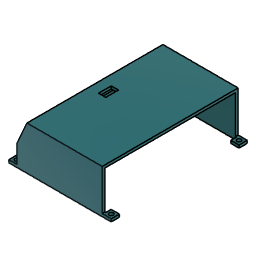
PerryBot (Autodesk Fusion 360 archive; units mm, degrees)
design "PerryBot2_Lid"
Autodesk Fusion 360 part; units mm, degrees
sketch "Sketch1" plane through (0, 0, 0) normal (0, 0, 1) x (1, 0, 0)
  line L0 (56.5, 75) -> (-56.5, 75)
  line L1 (-56.5, 75) -> (-56.5, -75)
  line L2 (-56.5, -75) -> (56.5, -75)
  line L3 (56.5, -75) -> (56.5, 75)
  line L4 (56.5, 75) -> (-56.5, -75) construction
  line L5 (-56.5, 75) -> (56.5, -75) construction
  line L6 (47.5, 75) -> (47.5, -75)
  line L7 (47.5, 66) -> (56.5, 66)
  line L8 (56.5, -66) -> (47.5, -66)
  dimension "d1" = 113
  dimension "d2" = 150
  dimension "d5" = 104
  dimension "d43" = 9
  dimension "d45" = 9
  constraint horizontal L0
  constraint perpendicular L0 L1
  constraint parallel L0 L2
  constraint parallel L1 L3
  constraint coincident L4 origin
  constraint coincident L5 origin
  constraint coincident L0 L6.start
  constraint coincident L2 L6.end
  constraint perpendicular L2 L6
  constraint coincident L6 L7.start
  constraint coincident L3 L7.end
  constraint perpendicular L6 L7
  constraint coincident L3 L8.start
  constraint coincident L6 L8.end
  constraint perpendicular L6 L8
  measures "d1" distance of L0.start L0.end
  measures "d2" distance of L0.start L2.end
  measures "d5" distance of L1 L6
  measures "d43" distance of L0 L7
  measures "d45" distance of L2 L8
extrude "Extrude1" add sketch "Sketch1" along normal blind 3 contours L0 L3 L6 L7 | L0 L1 L2 L6 | L2 L3 L6 L8 makes body 1
sketch "Sketch2" plane through (0, 0, 3) normal (0, 0, 1) x (-1, 0, 0)
  line L0 (-56.5, -66) -> (-56.5, -75)
  line L1 (-56.5, -75) -> (56.5, -75)
  line L2 (56.5, -75) -> (56.5, 75)
  line L3 (56.5, 75) -> (-56.5, 75)
  circle A0 centre (52, -70.5) radius 2.25
  line L4 (52, -70.5) -> (52, -75) construction
  line L5 (52, -70.5) -> (56.5, -70.5) construction
  line L6 (56.5, -75) -> (47.5, -75)
  line L7 (47.5, -75) -> (47.5, -66)
  line L8 (47.5, -66) -> (56.5, -66)
  line L9 (56.5, -66) -> (56.5, -75)
  line L10 (56.5, -75) -> (47.5, -66) construction
  line L11 (47.5, -75) -> (56.5, -66) construction
  line L12 (-47.5, -66) -> (-56.5, -66)
  line L13 (-56.5, 75) -> (-56.5, 66)
  line L14 (-56.5, 66) -> (-47.5, 66)
  line L15 (-47.5, 66) -> (-47.5, -66)
  point P0 (52, -70.5)
  dimension "d8" = 4.5
  dimension "d10" = 4.5
  constraint coincident P0 A0.centre
  constraint coincident L1 L4.end
  constraint perpendicular L1 L4
  constraint coincident L2 L5.end
  constraint perpendicular L2 L5
  constraint equal L4 L5
  constraint horizontal L6
  constraint perpendicular L6 L7
  constraint parallel L6 L8
  constraint parallel L7 L9
  constraint coincident L10 P0
  constraint coincident L11 P0
  constraint coincident L1.end L2.start
  measures "d8" diameter of A0
  measures "d10" distance of P0 L4.end
ref_plane "WorkPlane1" through (0, 0, 1.5) normal (0, 1, 0) x (-1, 0, 0)
ref_plane "WorkPlane2" through (0, 0, 1.5) normal (-1, 0, 0) x (0, -1, 0)
extrude "Extrude2" cut sketch "Sketch2" against normal blind 3 contours A0 bodies 1
mirror "Mirror1" about plane through (0, 0, 1.5) normal (-1, 0, 0) of "Extrude2"
mirror "Mirror2" about plane through (0, 0, 1.5) normal (0, 1, 0) of "Extrude2", "Mirror1"
ref_plane "WorkPlane3" through (0, -75, 1.5) normal (0, -1, 0) x (1, 0, 0)
sketch "Sketch5" plane through (0, -75, 0) normal (0, -1, 0) x (-1, 0, 0)
  line L0 (56.5, -3) -> (36.5, -3) construction
  line L1 (36.5, -3) -> (36.5, -48) construction
  line L2 (56.5, -3) -> (56.5, 0) construction
  line L3 (36.5, -48) -> (56.5, -3)
  line L4 (36.5, -48) -> (-46.5, -48)
  line L5 (-46.5, -48) -> (-46.5, -3)
  line L6 (-46.5, -3) -> (56.5, -3)
  line L7 (23, -104) -> (21.5469, -104)
  point P0 (56.5, 0)
  dimension "d32" = 20
  dimension "d33" = 45
  dimension "d34" = 3
  dimension "d36" = 83
  constraint horizontal L0
  constraint perpendicular L0 L1
  constraint coincident P0 L2.end
  constraint vertical L2
  constraint perpendicular L1 L4
  constraint perpendicular L0 L5
  constraint parallel L0 L6
  constraint perpendicular L5 L7
  measures "d32" distance of L0.start L0.end
  measures "d33" distance of L0.end L1.end
  measures "d34" distance of L0.start P0
  measures "d36" distance of L1.end L4.end
extrude "Extrude5" add sketch "Sketch5" against normal up to surface (150 mm away) separate body makes body 2
extrude "Extrude6" cut sketch "Sketch2" along normal blind 45 contours L1 L2 L6 L7 L8 L9 | A0 bodies 2
mirror "Mirror3" about plane through (0, 0, 1.5) normal (0, 1, 0) of "Extrude6"
sketch "Sketch7" plane through (46.5, 0, 0) normal (1, 0, 0) x (0, 1, 0)
  line L0 (75, 3) -> (75, 48)
  line L1 (75, 48) -> (-75, 48)
  line L2 (-75, 48) -> (-75, 3)
  line L3 (-75, 3) -> (75, 3)
  line L4 (-66, 0) -> (-72, 0)
  line L5 (-72, 0) -> (-72, 3)
  line L6 (-72, 3) -> (-66, 3)
  line L7 (-66, 3) -> (-66, 0)
  line L8 (-72, 3) -> (-72, 45)
  line L9 (-72, 45) -> (72, 45)
  line L10 (72, 45) -> (72, 3)
  dimension "d47" = 3
  dimension "d48" = 3
  dimension "d49" = 3
  constraint horizontal L4
  constraint vertical L5
  constraint horizontal L6
  constraint vertical L7
  constraint coincident L3 L5.end
  constraint perpendicular L6 L8
  constraint perpendicular L8 L9
  constraint coincident L3 L10.end
  constraint perpendicular L3 L10
  measures "d47" distance of L2.end L5.end
  measures "d48" distance of L1 L8.end
  measures "d49" distance of L0 L9.end
extrude "Extrude7" cut sketch "Sketch7" 1 faces at (47.5, 22, 1) against normal blind 83 contours L3 L6 L8 L9 L10 on bodies 1 bodies 1 2
sketch "Sketch8" plane through (0, 0, 3) normal (0, 0, 1) x (-1, 0, 0)
  circle A0 centre (52, -70.5) radius 2.25
  circle A1 centre (-52, -70.5) radius 2.25
  circle A2 centre (52, 70.5) radius 2.25
  circle A3 centre (-52, 70.5) radius 2.25
  line L0 (35.5, -66) -> (-56.5, -66)
  line L1 (-56.5, -66) -> (-56.5, -75)
  line L2 (-56.5, -75) -> (56.5, -75)
  line L3 (56.5, -75) -> (56.5, 75)
  line L4 (56.5, 75) -> (-56.5, 75)
  line L5 (-56.5, 75) -> (-56.5, 66)
  line L6 (-56.5, 66) -> (35.5, 66)
  line L7 (35.5, 66) -> (35.5, -66)
  line L8 (-47.5, 72) -> (-47.5, 66)
  line L9 (-47.5, 72) -> (35.5, 72)
  line L10 (35.5, 72) -> (35.5, 66)
  line L11 (-47.5, 66) -> (35.5, 66)
  line L12 (36.5, 72) -> (-46.5, 72)
  dimension "d52" = 9
  constraint coincident L6 L8.end
  constraint perpendicular L6 L8
  constraint perpendicular L3 L9
  constraint coincident L6.end L7.start
  constraint collinear L7 L10
  constraint collinear L9 L12
  measures "d52" distance of L5 L8
extrude "Extrude8" cut sketch "Sketch8" against normal up to surface (3 mm away) contours L6 L8 L9 L10 L11 L12 bodies 1
mirror "Mirror4" about plane through (0, 0, 1.5) normal (0, 1, 0) of "Extrude8"
sketch "Sketch9" plane through (0, -75, 0) normal (0, -1, 0) x (1, 0, 0)
  line L0 (-47.5, 23.25) -> (-47.5, 3)
  line L1 (-47.5, 3) -> (46.5, 3)
  line L2 (46.5, 3) -> (46.5, 48)
  line L3 (46.5, 48) -> (-36.5, 48)
  line L4 (-36.5, 48) -> (-47.5, 23.25)
  line L5 (-45.5, 3) -> (-45.5, 22.8256)
  line L6 (-45.5, 22.8256) -> (-36.5, 43.0756)
  line L7 (-41.3061, 32.2618) -> (-43.1338, 33.074) construction
  line L8 (-45.5, 16.8092) -> (-47.5, 16.8092) construction
  line L9 (-36.5, 43.0756) -> (-36.5, 3)
  dimension "d60" = 2
  constraint coincident L1 L5.start
  constraint perpendicular L1 L5
  constraint parallel L4 L6
  constraint vertical L3.end L6.end
  constraint coincident L6 L7.start
  constraint coincident L4 L7.end
  constraint perpendicular L4 L7
  constraint coincident L5 L8.start
  constraint coincident L0 L8.end
  constraint perpendicular L0 L8
  constraint equal L7 L8
  constraint coincident L1 L9.end
  constraint perpendicular L1 L9
  measures "d60" distance of L0 L5
extrude "Extrude9" cut sketch "Sketch9" against normal up to surface (144 mm away) from surface at -3 contours L1 L5 L6 L9 bodies 2
sketch "Sketch10" plane through (0, 0, 3) normal (0, 0, 1) x (-1, 0, 0)
  circle A0 centre (52, -70.5) radius 2.25
  circle A1 centre (-52, -70.5) radius 2.25
  circle A2 centre (52, 70.5) radius 2.25
  circle A3 centre (-52, 70.5) radius 2.25
  line L0 (35.5, 72) -> (35.5, -72)
  line L1 (35.5, -72) -> (-47.5, -72)
  line L2 (-47.5, -72) -> (-47.5, -66)
  line L3 (-47.5, -66) -> (-56.5, -66)
  line L4 (-56.5, -66) -> (-56.5, -75)
  line L5 (-56.5, -75) -> (56.5, -75)
  line L6 (56.5, -75) -> (56.5, 75)
  line L7 (56.5, 75) -> (-56.5, 75)
  line L8 (-56.5, 75) -> (-56.5, 66)
  line L9 (-56.5, 66) -> (-47.5, 66)
  line L10 (-47.5, 66) -> (-47.5, 72)
  line L11 (-47.5, 72) -> (35.5, 72)
  line L12 (35.5, 72) -> (45.5, 72)
  line L13 (45.5, 72) -> (45.5, -72)
  line L14 (45.5, -72) -> (35.5, -72)
  line L15 (35.5, 72) -> (35.5, -72)
  line L16 (45.5, -72) -> (45.5, 72)
  constraint coincident L0.start L11.end
  constraint perpendicular L5 L13
  constraint coincident L0.end L1.start
  constraint parallel L1 L14
  constraint collinear L13 L16
extrude "Extrude10" cut sketch "Sketch10" against normal blind 3 contours L0 L12 L13 L14 L15 L16 bodies 1
combine "Combine1" operation add target body 1 tool bodies 2
sketch "Sketch11" plane through (0, 0, 48) normal (0, 0, 1) x (-1, 0, 0)
  line L0 (-46.5, -75) -> (36.5, -75)
  line L1 (36.5, -75) -> (36.5, 75)
  line L2 (36.5, 75) -> (-46.5, 75)
  line L3 (-46.5, 75) -> (-46.5, -75)
  line L4 (17.5, -7) -> (25.5, -7)
  line L5 (25.5, -7) -> (25.5, 7)
  line L6 (25.5, 7) -> (17.5, 7)
  line L7 (17.5, 7) -> (17.5, -7)
  line L8 (17.5, -7) -> (25.5, 7) construction
  line L9 (25.5, -7) -> (17.5, 7) construction
  line L10 (36.5, 0) -> (-46.5, 0) construction
  point P0 (21.5, 0)
  dimension "d66" = 8
  dimension "d67" = 14
  dimension "d70" = 15
  constraint horizontal L4
  constraint perpendicular L4 L5
  constraint parallel L4 L6
  constraint parallel L5 L7
  constraint midpoint L1 L10.start
  constraint midpoint L3 L10.end
  constraint midpoint L8 P0
  constraint coincident L10 P0
  measures "d66" distance of L4.start L4.end
  measures "d67" distance of L4.start L6.end
  measures "d70" distance of L1 P0
extrude "Extrude11" cut sketch "Sketch11" against normal blind 3 contours L4 L5 L6 L7 bodies 1
sketch "Sketch12" plane through (0, -75, 0) normal (0, -1, 0) x (1, 0, 0)
  line L0 (-56.5, 0) -> (56.5, 0)
  line L1 (56.5, 0) -> (56.5, 3)
  line L2 (56.5, 3) -> (46.5, 3)
  line L3 (46.5, 3) -> (46.5, 48)
  line L4 (46.5, 48) -> (-36.5, 48)
  line L5 (-36.5, 48) -> (-47.5, 23.25)
  line L6 (-47.5, 23.25) -> (-47.5, 3)
  line L7 (-47.5, 3) -> (-56.5, 3)
  line L8 (-56.5, 3) -> (-56.5, 0)

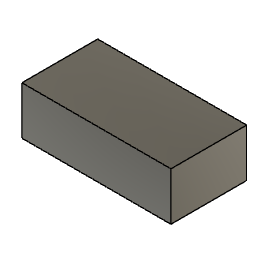
design "Lumenier_700mAh_3s_75c"
Autodesk Fusion 360 part; units mm, degrees
sketch "Sketch1" plane through (0, 0, 0) normal (0, 0, 1) x (1, 0, 0)
  line L0 (0, 0) -> (-59, 0)
  line L1 (-59, 0) -> (-59, 30)
  line L2 (-59, 30) -> (0, 30)
  line L3 (0, 30) -> (0, 0)
  dimension "d1" = 59
  dimension "d2" = 30
  constraint horizontal L0
  constraint vertical L1
  constraint horizontal L2
  constraint vertical L3
  constraint coincident L0.start L3.end
  measures "d1" distance of L1.end L2.end
  measures "d2" distance of L0.start L2.end
extrude "Extrude1" add sketch "Sketch1" along normal blind 19
sketch "Sketch2" plane through (-59, 0, 0) normal (-1, 0, 0) x (0, -1, 0)
  line L0 (-30, 0) -> (0, 0)
  line L1 (0, 0) -> (0, 19)
  line L2 (0, 19) -> (-30, 19)
  line L3 (-30, 19) -> (-30, 0)
  line L4 (-30, 0) -> (-22, 0)
  line L5 (-22, 0) -> (-22, 8)
  line L6 (-22, 8) -> (-30, 8)
  line L7 (-30, 8) -> (-30, 0)
  dimension "d5" = 8
  dimension "d6" = 8
  constraint horizontal L4
  constraint vertical L5
  constraint horizontal L6
  constraint vertical L7
  constraint coincident L0.start L3.end
  measures "d5" distance of L5.end L6.end
  measures "d6" distance of L4.end L5.end
extrude "Extrude2" add sketch "Sketch2" along normal blind 5 contours L0 L3 L4 L5 L6 L7

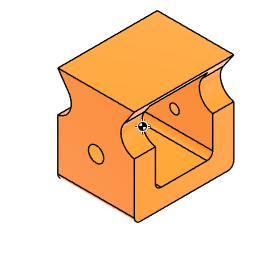
design "PerryBot2_Spinner"
Autodesk Fusion 360 part; units mm, degrees
sketch "Sketch1" plane through (0, 0, 0) normal (1, 0, 0) x (0, 1, 0)
  line L0 (-26, -12) -> (26, -12)
  line L1 (26, -12) -> (26, -22)
  line L2 (26, -22) -> (-26, -22)
  line L3 (-26, -22) -> (-26, -12)
  line L4 (-26, 29) -> (26, 29)
  line L5 (26, 29) -> (26, 25)
  line L6 (26, 25) -> (-26, 25)
  line L7 (-26, 25) -> (-26, 29)
  line L8 (0, 25) -> (0, -12) construction
  line L9 (-26, 25) -> (-15, 25)
  line L10 (-15, 25) -> (-15, -12)
  line L11 (-15, -12) -> (-26, -12)
  line L12 (-26, -12) -> (-26, 25)
  line L13 (26, 25) -> (15, 25)
  line L14 (15, 25) -> (15, -12)
  line L15 (15, -12) -> (26, -12)
  line L16 (26, -12) -> (26, 25)
  dimension "d4" = 11
  dimension "d5" = 52
  dimension "d6" = 4
  dimension "d7" = 10
  dimension "d8" = 12
  dimension "d9" = 25
  constraint horizontal L0
  constraint vertical L1
  constraint horizontal L2
  constraint vertical L3
  constraint horizontal L4
  constraint vertical L5
  constraint horizontal L6
  constraint vertical L7
  constraint midpoint L6 L8.start
  constraint midpoint L0 L8.end
  constraint coincident origin L8
  constraint equal L0 L4
  constraint horizontal L9
  constraint vertical L10
  constraint horizontal L11
  constraint vertical L12
  constraint coincident L0 L10.end
  constraint horizontal L13
  constraint vertical L14
  constraint horizontal L15
  constraint vertical L16
  constraint coincident L0 L14.end
  constraint symmetric L8 L10 L14
  constraint symmetric L8 L12 L16
  measures "d4" distance of L6.end L9.end
  measures "d5" distance of L4.start L4.end
  measures "d6" distance of L4.end L5.end
  measures "d7" distance of L0.end L1.end
  measures "d8" distance of origin L0
  measures "d9" distance of origin L6
extrude "Extrude1" add sketch "Sketch1" along normal mid plane 40 contours L0 L6 L9 L10 L11 L12 | L0 L1 L2 L3 L11 L15 | L4 L5 L6 L7 L9 L13 | L0 L6 L13 L14 L15 L16 makes body 1
sketch "Sketch2" plane through (0, 26, 0) normal (0, 1, 0) x (-1, 0, 0)
  line L0 (20, 29) -> (-20, 29)
  line L1 (-20, 29) -> (-20, -22)
  line L2 (-20, -22) -> (20, -22)
  line L3 (20, -22) -> (20, 29)
  circle A0 centre (0, 0) radius 2.45
  dimension "d13" = 4.9
  constraint coincident A0.centre origin
  measures "d13" diameter of A0
extrude "Extrude2" cut sketch "Sketch2" against normal up to surface (11 mm away) contours A0 bodies 1
sketch "Sketch3" plane through (0, 26, 0) normal (0, 1, 0) x (-1, 0, 0)
  circle A0 centre (0, 0) radius 2.45
  line L0 (20, 29) -> (-20, 29)
  line L1 (-20, 29) -> (-20, -22)
  line L2 (-20, -22) -> (20, -22)
  line L3 (20, -22) -> (20, 29)
  circle A1 centre (0, 0) radius 14.5
  dimension "d17" = 29
  constraint coincident A0.centre A1.centre
  measures "d17" diameter of A1
extrude "Extrude3" cut sketch "Sketch3" against normal blind 6 contours A1 bodies 1
sketch "Sketch4" plane through (0, 26, 0) normal (0, 1, 0) x (-1, 0, 0)
  circle A0 centre (0, 0) radius 14.5
  line L0 (20, 29) -> (-20, 29)
  line L1 (-20, 29) -> (-20, -22)
  line L2 (-20, -22) -> (20, -22)
  line L3 (20, -22) -> (20, 29)
  line L4 (0, 0) -> (20, 29) construction
  line L5 (0, 0) -> (-20, 29) construction
  line L6 (20, 29) -> (14.4828, 21)
  line L7 (0, 0) -> (0, 29) construction
  line L8 (-20, 29) -> (-14.4828, 21)
  arc A1 (14.4828, 21) -> (20, 7.8041) centre (21.4801, 16.1743) ccw
  arc A2 (-20, 7.8041) -> (-14.4828, 21) centre (-21.4801, 16.1743) ccw
  dimension "d20" = 8
  dimension "d21" = 8.5
  constraint coincident A0.centre L4.start
  constraint coincident L0.start L3.end
  constraint coincident L0.end L1.start
  constraint coincident L4 L6.end
  constraint parallel L4 L6
  constraint vertical L7
  constraint symmetric L0.start L7 L0.end
  constraint symmetric L6.end L7 L8.end
  constraint coincident L3 A1.end
  constraint tangent L6 A1
  constraint symmetric L7 A1.end A2.start
  constraint symmetric L7 A1 A2
  constraint coincident L0 L7.end
  measures "d20" vertical distance of L0.start L6.end
  measures "d21" radius of A1
extrude "Extrude4" cut sketch "Sketch4" against normal blind 80 contours L3 L6 A1 | L1 L8 A2 bodies 1
fillet "Fillet1" radius 3 4 edges at (0, 15, -12) (0, -15, -12) (0, 26, -22) (0, -26, -22) on bodies 1
sketch "Sketch5" plane through (0, -26, 0) normal (0, -1, 0) x (1, 0, 0)
  line L0 (-20, -19) -> (20, -19)
  line L1 (20, -19) -> (20, 7.8041)
  arc A0 (14.4828, 21) -> (20, 7.8041) centre (21.4801, 16.1743) ccw
  line L2 (14.4828, 21) -> (20, 29)
  line L3 (20, 29) -> (-20, 29)
  line L4 (-20, 29) -> (-14.4828, 21)
  arc A1 (-20, 7.8041) -> (-14.4828, 21) centre (-21.4801, 16.1743) ccw
  line L5 (-20, 7.8041) -> (-20, -19)
  circle A2 centre (0, 0) radius 4
  dimension "d32" = 8
  constraint coincident A2.centre origin
  measures "d32" diameter of A2
sketch "Sketch6" plane through (0, 0, 0) normal (1, 0, 0) x (0, 1, 0)
  line L0 (0, 0) -> (-26, 0)
  line L1 (-26, 0) -> (-26, 38)
  line L2 (-26, 38) -> (0, 38)
  line L3 (26, 0) -> (26, 38)
  line L4 (26, 38) -> (0, 38)
  line L5 (0, 0) -> (26, 0)
  dimension "d28" = 26
  dimension "d29" = 38
  dimension "d31" = 26
  constraint horizontal L0
  constraint vertical L1
  constraint horizontal L2
  constraint coincident L0.start L5.start
  constraint equal L2 L4
  constraint equal L1 L3
  constraint equal L0 L5
  constraint horizontal L4
  constraint horizontal L5
  constraint vertical L3
  constraint coincident L2.end L4.end
  measures "d28" distance of L0.start L0.end
  measures "d29" distance of L0.end L1.end
  measures "d31" distance of L3.end L2.end
revolve "Revolve1" add sketch "Sketch6" angle 360 about axis through (0, 21.5, 0) along (0, -1, 0) separate body makes body 2
extrude "Extrude5" cut sketch "Sketch5" against normal blind 11 contours A2 bodies 1
sketch "Sketch7" plane through (0, 20, 0) normal (0, 1, 0) x (-1, 0, 0)
  circle A0 centre (0, 0) radius 2.45
  circle A1 centre (0, 0) radius 14.5
  line L0 (0, 0) -> (0, 14.5) construction
  line L1 (0, 1.75) -> (0, 22.5) construction
  line L2 (-2.7394, 11.5) -> (2.7394, 11.5)
  line L3 (3.4794, 9.8273) -> (0.7399, 6.8139)
  line L4 (-0.7399, 6.8139) -> (-3.4794, 9.8273)
  arc A2 (-2.7394, 11.5) -> (-3.4794, 9.8273) centre (-2.7394, 10.5) ccw
  arc A3 (3.4794, 9.8273) -> (2.7394, 11.5) centre (2.7394, 10.5) ccw
  arc A4 (-0.7399, 6.8139) -> (0.7399, 6.8139) centre (0, 7.4866) ccw
  arc A5 (-11.7837, 0.9483) -> (-10.4215, -0.2723) centre (-10.8326, 0.6393) ccw
  line L5 (-6.7091, 1.4019) -> (-10.4215, -0.2723)
  arc A6 (-6.7091, 1.4019) -> (-6.2518, 2.8093) centre (-7.1202, 2.3135) ccw
  arc A7 (-8.2712, 6.3459) -> (-10.0906, 6.1591) centre (-9.1396, 5.85) ccw
  line L6 (-8.2712, 6.3459) -> (-6.2518, 2.8093)
  line L7 (-11.7837, 0.9483) -> (-10.0906, 6.1591)
  arc A8 (-4.5433, -10.9139) -> (-2.9615, -9.9956) centre (-3.9555, -10.1049) ccw
  line L8 (-3.4065, -5.9475) -> (-2.9615, -9.9956)
  arc A9 (-3.4065, -5.9475) -> (-4.6038, -5.0777) centre (-4.4005, -6.0568) ccw
  arc A10 (-8.5912, -5.9053) -> (-8.9758, -7.6935) centre (-8.388, -6.8845) ccw
  line L9 (-8.5912, -5.9053) -> (-4.6038, -5.0777)
  line L10 (-4.5433, -10.9139) -> (-8.9758, -7.6935)
  arc A11 (8.9758, -7.6935) -> (8.5912, -5.9053) centre (8.388, -6.8845) ccw
  line L11 (4.6038, -5.0777) -> (8.5912, -5.9053)
  arc A12 (4.6038, -5.0777) -> (3.4065, -5.9475) centre (4.4005, -6.0568) ccw
  arc A13 (2.9615, -9.9956) -> (4.5433, -10.9139) centre (3.9555, -10.1049) ccw
  line L12 (2.9615, -9.9956) -> (3.4065, -5.9475)
  line L13 (8.9758, -7.6935) -> (4.5433, -10.9139)
  arc A14 (10.0906, 6.1591) -> (8.2712, 6.3459) centre (9.1396, 5.85) ccw
  line L14 (6.2518, 2.8093) -> (8.2712, 6.3459)
  arc A15 (6.2518, 2.8093) -> (6.7091, 1.4019) centre (7.1202, 2.3135) ccw
  arc A16 (10.4215, -0.2723) -> (11.7837, 0.9483) centre (10.8326, 0.6393) ccw
  line L15 (10.4215, -0.2723) -> (6.7091, 1.4019)
  line L16 (10.0906, 6.1591) -> (11.7837, 0.9483)
  point P0 (-5, 11.5)
  point P1 (5, 11.5)
  point P2 (0, 6)
  point P3 (-5.7063, 1.8541)
  point P4 (-3.5267, -4.8541)
  point P5 (3.5267, -4.8541)
  point P6 (5.7063, 1.8541)
  dimension "d38" = 5.5
  dimension "d39" = 10
  dimension "d40" = 3
  dimension "d41" = 1
  dimension "d43" = 360
  constraint coincident A0.centre A1.centre
  constraint coincident A1 L0.end
  constraint horizontal L2
  constraint symmetric L0 L3 L4
  constraint vertical L0
  constraint coincident P0 L2
  constraint coincident P0 L4
  constraint tangent L2 A2
  constraint tangent L4 A2
  constraint coincident P1 L2
  constraint coincident P1 L3
  constraint tangent L2 A3
  constraint tangent L3 A3
  constraint equal A2 A3
  constraint coincident P2 L3
  constraint coincident P2 L4
  constraint tangent L3 A4
  constraint tangent L4 A4
  constraint equal A2 A4
  measures "d38" distance of L2 P2
  measures "d39" distance of P0 P1
  measures "d40" distance of L0.end L2
  measures "d41" radius of A2
extrude "Extrude6" add sketch "Sketch7" along normal blind 2.5 contours L2 L3 L4 A2 A3 A4 | A5 L5 A6 A7 L6 L7 | A8 L8 A9 A10 L9 L10 | A11 L11 A12 A13 L12 L13 | A14 L14 A15 A16 L15 L16 bodies 1
fillet "Fillet2" radius 0.5 5 faces at (0.2466, 22.5, 9.938) (9.5278, 22.5, 2.8364) (6.0409, 22.5, -7.895) (-6.0409, 22.5, -7.895) (-9.5278, 22.5, 2.8364) on bodies 1
fillet "Fillet3" radius 0.5 1 edges at (13.5187, 26, 5.2434) on bodies 1
hidden bodies 2
